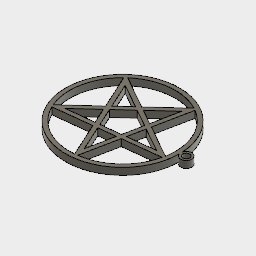
cld9 (Autodesk Fusion 360 design; units mm, degrees)
Autodesk Fusion 360 part; units mm, degrees
sketch "草图1" plane through (0, 0, 0) normal (0, 1, 0) x (1, 0, 0)
  line L0 (16.2048, 31.9119) -> (3.5265, -30.6998)
  line L1 (15.1919, 26.9095) -> (-28.1075, -12.8407)
  line L2 (-28.1075, -12.8407) -> (30.287, -6.1328)
  line L3 (-20.8979, 22.7638) -> (30.287, -6.1328)
  circle A0 centre (0, 0) radius 40.5463
  circle A1 centre (0, 0) radius 37.5463
  line L4 (-20.8979, 22.7638) -> (3.5265, -30.6998)
  line L5 (-4.0939, 13.277) -> (-34.5546, -14.6869)
  line L6 (-36.8886, -16.8296) -> (-36.9379, -16.8748)
  line L7 (-36.9379, -16.8748) -> (-36.8714, -16.8672)
  line L8 (4.6067, -40.2838) -> (4.6345, -40.3446)
  line L9 (4.6477, -40.2791) -> (4.6345, -40.3446)
  line L10 (-33.7238, -16.5056) -> (36.588, -8.4287)
  line L11 (39.7357, -8.0672) -> (39.8021, -8.0595)
  line L12 (39.7439, -8.0267) -> (39.8021, -8.0595)
  line L13 (19.9646, 35.3635) -> (19.9513, 35.298)
  line L14 (19.3225, 32.1926) -> (5.2765, -37.1737)
  line L15 (19.9646, 35.3635) -> (19.9154, 35.3183)
  line L16 (17.5814, 33.1756) -> (-1.7702, 15.4103)
  line L17 (-27.4633, 29.9154) -> (-27.4355, 29.8546)
  line L18 (-26.119, 26.9727) -> (3.2901, -37.4019)
  line L19 (-27.4633, 29.9154) -> (-27.4051, 29.8825)
  line L20 (-24.646, 28.3249) -> (36.9848, -6.469)
  dimension "d3" = 3
extrude "拉伸1" add sketch "草图1" along normal blind 5 contours L0 A1 L14 L16 L20 | L0 L1 L16 L20 | L1 L3 A1 L4 L5 L18 L20 | L0 L3 L14 L20 | L0 L1 L3 L20 | L0 L2 L3 L14 | L2 L3 A1 L10 L14 L20 | L1 L3 L4 L5 | L0 L2 L10 L14 | L0 L2 L4 L10 | L1 L2 L4 L18 | L1 L4 L5 L18 | L1 L2 A1 L5 L10 L18 | L0 A1 L4 L10 L14 L18 | L2 L4 L10 L18 | A0 makes body 1
torus "圆环体基本要素1" add centre line diameter 8 section diameter 5 placed x (1, 0, 0) y (0, 0, -1) z (0, 1, 0) at (42.5101, 0, -38.453) separate body makes body 2
delete_face "删除面1" 1 faces at (48.9525, -0.4954, -38.1315) on bodies 2
sketch "草图3" plane through (0, 0, 0) normal (0, 1, 0) x (1, 0, 0)
  circle A0 centre (53.2848, 1.0037) radius 2.5
  circle A1 centre (53.2848, 1.0037) radius 4
extrude "拉伸2" add sketch "草图3" along normal blind 5 separate body makes body 3
move_body "移动1" bodies 3 to x (1, 0, 0) y (0, 1, 0) z (0, 0, 1) at (-9, 0, 0)
combine "合并1" operation add target body 1 tool bodies 3
